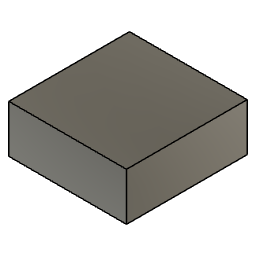
Block (Autodesk Fusion 360 design; units mm, degrees)
Autodesk Fusion 360 part; units mm, degrees
sketch "Sketch1" plane through (0, 0, 0) normal (0, 0, 1) x (1, 0, 0)
  line L0 (-49.4163, 50.658) -> (0, 50.658)
  line L1 (0, 50.658) -> (0, 0)
  line L2 (0, 0) -> (-49.4163, 0)
  line L3 (-49.4163, 0) -> (-49.4163, 50.658)
  constraint horizontal L0
  constraint vertical L1
  constraint horizontal L2
  constraint vertical L3
  constraint coincident L1.end L2.start
extrude "Extrude1" add sketch "Sketch1" along normal blind 20
